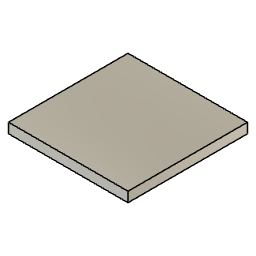
final_assembly v4 (Autodesk Fusion 360 archive; units mm, degrees)
design "solar_cell"
Autodesk Fusion 360 part; units mm, degrees
sketch "Sketch1" plane through (0, 0, 0) normal (0, 0, 1) x (1, 0, 0)
  line L0 (-60, 60) -> (0, 60)
  line L1 (0, 60) -> (0, 0)
  line L2 (0, 0) -> (-60, 0)
  line L3 (-60, 0) -> (-60, 60)
  dimension "d1" = 60
  dimension "d2" = 60
  constraint horizontal L0
  constraint vertical L1
  constraint horizontal L2
  constraint vertical L3
  constraint coincident L1.end L2.start
  measures "d1" distance of L0.start L2.end
  measures "d2" distance of L0.start L0.end
extrude "Extrude1" add sketch "Sketch1" along normal blind 5

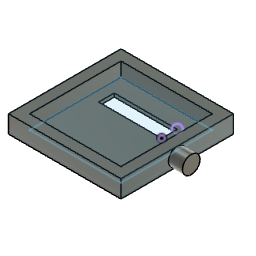
design "solar_cell_holder"
Autodesk Fusion 360 part; units mm, degrees
sketch "Sketch1" plane through (0, 0, 0) normal (0, 0, 1) x (1, 0, 0)
  line L0 (-80, 80) -> (0, 80)
  line L1 (0, 80) -> (0, 0)
  line L2 (0, 0) -> (-80, 0)
  line L3 (-80, 0) -> (-80, 80)
  line L4 (-65.1867, 49.3204) -> (-20.3412, 49.3204)
  line L5 (-20.3412, 49.3204) -> (-20.3412, 60.4169)
  line L6 (-20.3412, 60.4169) -> (-65.1867, 60.4169)
  line L7 (-65.1867, 60.4169) -> (-65.1867, 49.3204)
  dimension "d1" = 80
  dimension "d2" = 80
  constraint horizontal L0
  constraint vertical L1
  constraint horizontal L2
  constraint vertical L3
  constraint horizontal L4
  constraint vertical L5
  constraint horizontal L6
  constraint vertical L7
  constraint coincident L1.end L2.start
  measures "d1" distance of L0.start L2.end
  measures "d2" distance of L0.start L0.end
extrude "Extrude1" add sketch "Sketch1" along normal blind 2.5
sketch "Sketch2" plane through (0, 0, 2.5) normal (0, 0, 1) x (-1, 0, 0)
  line L0 (65.1867, -60.4169) -> (20.3412, -60.4169)
  line L1 (65.1867, -49.3204) -> (65.1867, -60.4169)
  line L2 (20.3412, -49.3204) -> (65.1867, -49.3204)
  line L3 (20.3412, -60.4169) -> (20.3412, -49.3204)
  line L4 (80, 0) -> (0, 0)
  line L5 (0, 0) -> (0, -80)
  line L6 (0, -80) -> (80, -80)
  line L7 (80, -80) -> (80, 0)
  line L8 (72.5, -72.5) -> (7.5, -72.5)
  line L9 (7.5, -72.5) -> (7.5, -7.5)
  line L10 (7.5, -7.5) -> (72.5, -7.5)
  line L11 (72.5, -7.5) -> (72.5, -72.5)
  dimension "d14" = 65
  constraint horizontal L8
  constraint vertical L9
  constraint horizontal L10
  constraint vertical L11
  measures "d14" distance of L8.end L9.end
extrude "Extrude3" add sketch "Sketch2" along normal blind 10 contours L4 L5 L6 L7
sketch "Sketch3" plane through (0, 0, 0) normal (1, 0, 0) x (0, 1, 0)
  line L0 (0, 0) -> (80, 0)
  line L1 (80, 0) -> (80, 12.5)
  line L2 (80, 12.5) -> (0, 12.5)
  line L3 (0, 12.5) -> (0, 0)
sketch "Sketch4" plane through (0, 0, 0) normal (1, 0, 0) x (0, 1, 0)
  circle A0 centre (40, 6.25) radius 6.25
  line L0 (80, 12.5) -> (0, 12.5)
  line L1 (0, 0) -> (80, 0)
  line L2 (40, 6.25) -> (80, 6.25) construction
  line L3 (40, 6.25) -> (0, 6.25) construction
  line L4 (0, 12.5) -> (0, 0)
  line L5 (80, 0) -> (80, 12.5)
  constraint tangent A0 L0
  constraint tangent A0 L1
  constraint coincident A0.centre L2.start
  constraint horizontal L2
  constraint parallel L2 L3
  constraint equal L2 L3
  constraint coincident L3.end L4
  constraint coincident L2.end L5
extrude "Extrude4" add sketch "Sketch4" along normal blind 10 contours A0
sketch "Sketch5" plane through (-80, 0, 0) normal (-1, 0, 0) x (0, -1, 0)
  line L0 (-80, 0) -> (0, 0)
  line L1 (0, 0) -> (0, 12.5)
  line L2 (0, 12.5) -> (-80, 12.5)
  line L3 (-80, 12.5) -> (-80, 0)
  line L4 (-40, 10.5531) -> (-55, 9)
  line L5 (-40.1118, 2.279) -> (-54.9402, 3.512)
  line L6 (-40, 10.5531) -> (-24.876, 8.9944)
  line L7 (-40.1118, 2.279) -> (-24.8941, 3.6094)
  arc A0 (-24.8941, 3.6094) -> (-24.876, 8.9944) centre (-25.1534, 6.3028) ccw
  arc A1 (-55, 9) -> (-54.9402, 3.512) centre (-54.7162, 6.2588) ccw
  constraint tangent L6 A0
  constraint tangent L4 A1
extrude "Extrude5" cut sketch "Sketch5" against normal blind 5 contours L4 L5 L6 L7 A0 A1
sketch "Sketch6" plane through (0, 0, 2.5) normal (0, 0, 1) x (-1, 0, 0)
sketch "Sketch7" plane through (0, 0, 12.5) normal (0, 0, 1) x (-1, 0, 0)
  line L0 (7.5, -7.5) -> (72.5, -7.5)
  line L1 (72.5, -7.5) -> (72.5, -72.5)
  line L2 (72.5, -72.5) -> (7.5, -72.5)
  line L3 (7.5, -72.5) -> (7.5, -7.5)
  line L4 (80, -80) -> (80, 0)
  line L5 (80, 0) -> (0, 0)
  line L6 (0, 0) -> (0, -40)
  line L7 (0, -40) -> (0, -80)
  line L8 (0, -80) -> (80, -80)
equation "width_solar_cell = 60 mm"
equation "height_solar_cell = 10 mm"
equation "length_solar_cell = 60 mm"

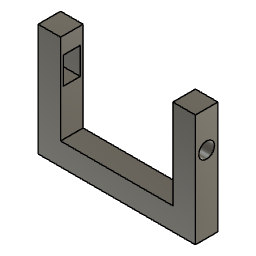
design "solar_bracket"
Autodesk Fusion 360 part; units mm, degrees
sketch "Sketch1" plane through (0, 0, 0) normal (0, 0, 1) x (1, 0, 0)
  line L0 (-50, 10) -> (50, 10)
  line L1 (50, 10) -> (50, -10)
  line L2 (50, -10) -> (-50, -10)
  line L3 (-50, -10) -> (-50, 10)
  dimension "d7" = 20
  dimension "d8" = 100
  constraint horizontal L0
  constraint vertical L1
  constraint horizontal L2
  constraint vertical L3
  measures "d7" distance of L0.start L2.end
  measures "d8" distance of L0.start L0.end
extrude "Extrude1" add sketch "Sketch1" along normal blind 20
sketch "Sketch2" plane through (50, 0, 0) normal (1, 0, 0) x (0, 1, 0)
  line L0 (-10, 0) -> (10, 0)
  line L1 (10, 0) -> (10, 20)
  line L2 (10, 20) -> (-10, 20)
  line L3 (-10, 20) -> (-10, 0)
  line L4 (-8, 8) -> (8, 8)
  line L5 (8, 8) -> (8, 2)
  line L6 (8, 2) -> (-8, 2)
  line L7 (-8, 2) -> (-8, 8)
  constraint horizontal L4
  constraint vertical L5
  constraint horizontal L6
  constraint vertical L7
extrude "Extrude2" cut sketch "Sketch2" against normal through all contours L4 L5 L6 L7
sketch "Sketch4" plane through (0, 0, 0) normal (0, 0, 1) x (1, 0, 0)
  line L0 (-70, 10) -> (-50, 10)
  line L1 (-50, 10) -> (-50, -10)
  line L2 (-50, -10) -> (-70, -10)
  line L3 (-70, -10) -> (-70, 10)
  line L4 (70, -10) -> (50, -10)
  line L5 (50, -10) -> (50, 10)
  line L6 (50, 10) -> (70, 10)
  line L7 (70, 10) -> (70, -10)
  line L8 (50, 10) -> (-50, 10)
  line L9 (-50, -10) -> (50, -10)
  dimension "d6" = 20
  constraint horizontal L0
  constraint vertical L1
  constraint horizontal L2
  constraint vertical L3
  constraint horizontal L4
  constraint vertical L5
  constraint horizontal L6
  constraint vertical L7
  constraint collinear L6 L8
  constraint collinear L2 L4
  constraint collinear L4 L9
  constraint collinear L0 L8
  constraint equal L2 L4
  constraint coincident L4.end L5.start
  constraint coincident L0.end L1.start
  measures "d6" distance of L4.start L4.end
extrude "Extrude3" add sketch "Sketch4" along normal blind 100 contours L0 L1 L2 L3 | L4 L5 L6 L7
sketch "Sketch5" plane through (-50, 0, 0) normal (1, 0, 0) x (0, 1, 0)
  line L0 (-10, 20) -> (10, 20)
  line L1 (10, 20) -> (10, 100)
  line L2 (10, 100) -> (-10, 100)
  line L3 (-10, 100) -> (-10, 20)
  line L4 (-7.5, 85) -> (7.5, 85)
  line L5 (7.5, 85) -> (7.5, 61)
  line L6 (7.5, 61) -> (-7.5, 61)
  line L7 (-7.5, 61) -> (-7.5, 85)
  line L8 (0, 85) -> (0, 100)
  dimension "d9" = 15
  dimension "d10" = 24
  dimension "d11" = 15
  constraint horizontal L4
  constraint vertical L5
  constraint horizontal L6
  constraint vertical L7
  constraint midpoint L4 L8.start
  constraint midpoint L2 L8.end
  constraint perpendicular L4 L8
  measures "d9" distance of L4.start L4.end
  measures "d10" distance of L4.end L5.end
  measures "d11" distance of L8.start L8.end
extrude "Extrude4" cut sketch "Sketch5" against normal blind 24 contours L4 L5 L6 L7
sketch "Sketch6" plane through (50, 0, 0) normal (-1, 0, 0) x (0, -1, 0)
  line L0 (-10, 20) -> (10, 20)
  line L1 (10, 20) -> (10, 100)
  line L2 (10, 100) -> (-10, 100)
  line L3 (-10, 100) -> (-10, 20)
  circle A0 centre (0, 68) radius 7
  line L4 (-10, 68) -> (0, 68) construction
  line L5 (0, 68) -> (10, 68) construction
  line L6 (0, 100) -> (0, 68) construction
  dimension "d24" = 14
  dimension "d25" = 32
  constraint coincident L3 L4.start
  constraint coincident A0.centre L4.end
  constraint perpendicular L3 L4
  constraint coincident L1 L5.end
  constraint perpendicular L1 L5
  constraint equal L4 L5
  constraint midpoint L2 L6.start
  measures "d24" diameter of A0
  measures "d25" distance of L6.start A0.centre
extrude "Extrude5" cut sketch "Sketch6" against normal through all contours A0
sketch "Sketch7" plane through (0, 0, 0) normal (0, 0, -1) x (1, 0, 0)
  line L0 (70, 10) -> (-70, 10)
  line L1 (-70, 10) -> (-70, -10)
  line L2 (-70, -10) -> (70, -10)
  line L3 (70, -10) -> (70, 10)
  line L4 (0, 4) -> (-15, 3)
  line L5 (0, 4) -> (14.5743, 2.8561)
  arc A0 (-15, 3) -> (-15, -3) centre (-14.8, 0) ccw
  line L6 (-15, -3) -> (0, -4.4941)
  line L7 (0, -4.4941) -> (15, -3)
  arc A1 (15, -3) -> (14.5743, 2.8561) centre (14.7089, -0.0777) ccw
  constraint tangent L4 A0
  constraint tangent L7 A1
extrude "Extrude6" cut sketch "Sketch7" against normal blind 2 contours L4 L5 A0 L6 L7 A1
equation "d25 = 26 mm + 6 mm"
